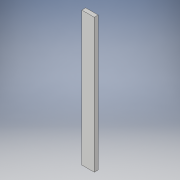
# Autodesk Inventor part: EastPole
Saved by Autodesk Inventor 2018 (Build 220112000, 112)
## iProperties
Created: 2019-04-28
Part Number: EastPole
Material: Generic
Document SubType Name: Modeling
Designer: snipe
Density: 1 g/cm^3
Appearance: Default
Author: snipe
Autodesk Inventor part; units mm, degrees
ref_plane "YZ Plane" through (0, 0, 0) normal (1, 0, 0) x (0, 1, 0)
ref_plane "XZ Plane" through (0, 0, 0) normal (0, 1, 0) x (-1, 0, 0)
ref_plane "XY Plane" through (0, 0, 0) normal (0, 0, 1) x (1, 0, 0)
sketch "Sketch1" plane through (0, 0, 0) normal (0, 1, 0) x (-1, 0, 0)
  line L0 (120.65, -38.1) -> (-120.65, -38.1)
  line L1 (-120.65, -38.1) -> (-120.65, 38.1)
  line L2 (-120.65, 38.1) -> (120.65, 38.1)
  line L3 (120.65, 38.1) -> (120.65, -38.1)
  line L4 (0, -53.34) -> (0, 53.34) projected
  line L5 (-168.91, 0) -> (168.91, 0) projected
  point P0 (0, 0)
  dimension "d0" = 241.3
  dimension "d1" = 76.2
  constraints: 8 end point, 2 parallel, 1 horizontal, 1 perpendicular, 2 other
  measures "d0" distance of L1.end L2.end
  measures "d1" distance of L0.end L1.end
extrude "Extrusion1" add sketch "Sketch1" along normal blind 2590.8
body "Solid1"
